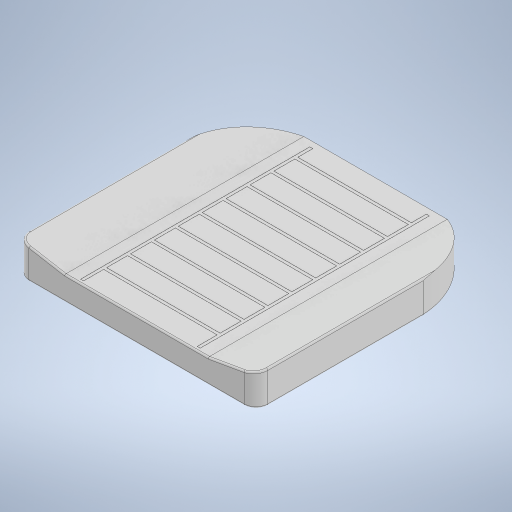
# Autodesk Inventor part: TheSeat(H)
Saved by Autodesk Inventor 2023 (Build 270158030, 158C)
## iProperties
Created: 2023-03-04
Part Number: TheSeat(H)
Material: Generic
Document SubType Name: Modeling
Designer: mpino
Density: 1 g/cm^3
Appearance: Default
Author: mpino
Autodesk Inventor part; units mm, degrees
ref_plane "YZ Plane" through (0, 0, 0) normal (1, 0, 0) x (0, 1, 0)
ref_plane "XZ Plane" through (0, 0, 0) normal (0, 1, 0) x (-1, 0, 0)
ref_plane "XY Plane" through (0, 0, 0) normal (0, 0, 1) x (1, 0, 0)
sketch "Sketch1" plane through (0, 0, 0) normal (0, 1, 0) x (-1, 0, 0)
  line L0 (0, 0) -> (508, 0)
  line L1 (508, 0) -> (508, -508)
  line L2 (508, -508) -> (0, -508)
  line L3 (0, -508) -> (0, 0)
  dimension "d0" = 508
  dimension "d1" = 508
  constraints: 8 end point, 2 parallel, 1 horizontal, 1 perpendicular
  measures "d0" distance of L1.end L2.end
  measures "d1" distance of L0.end L1.end
extrude "Extrusion1" add sketch "Sketch1" along normal blind 50.8
sketch "Sketch2" plane through (0, 50.8, 0) normal (0, 1, 0) x (1, 0, 0)
  line L0 (-508, 0) -> (0, 0) projected
  line L1 (0, 0) -> (0, 25.4)
  line L2 (0, 0) -> (-25.4, 0)
  arc A0 (-25.4, 0) -> (0, 25.4) centre (-25.4, 25.4) ccw
  line L3 (-508, 0) -> (-482.6, 0)
  line L4 (-482.6, 0) -> (-508, 0)
  line L5 (-508, 0) -> (-508, 25.4)
  arc A1 (-508, 25.4) -> (-482.6, 0) centre (-482.6, 25.4) ccw
  line L6 (0, 508) -> (0, 355.6)
  line L7 (0, 508) -> (-101.6, 508)
  arc A2 (0, 355.6) -> (-101.6, 508) centre (-177.6045, 347.2637) ccw
  line L8 (-508, 508) -> (-406.4, 508)
  line L9 (-508, 508) -> (-508, 355.6)
  arc A3 (-406.4, 508) -> (-508, 355.6) centre (-330.3955, 347.2637) ccw
  line L10 (0, 508) -> (-508, 508) projected
  point P0 (-7.4395, 7.4395)
  dimension "d11" = 25.4
  dimension "d12" = 25.4
  dimension "d13" = 25.4
  dimension "d14" = 25.4
  dimension "d81" = 152.4
  dimension "d83" = 177.8
  dimension "d85" = 152.4
  dimension "d86" = 177.8
  dimension "d88" = 7.4395
  dimension "d91" = 101.6
  dimension "d92" = 101.6
  constraints: 18 end point, 9 point on circle, 4 centre point, 4 point on line, 3 tangent, 2 vertical, 1 collinear
  measures "d11" distance of L0.end L1.end
  measures "d12" distance of L0.end L2.end
  measures "d13" distance of L0.start L3.end
  measures "d14" distance of L0.start L5.end
  measures "d81" distance of L6.start L6.end
  measures "d83" radius of A2
  measures "d85" distance of L8.start L9.end
  measures "d86" radius of A3
  measures "d88" distance from line of L1 point (-7.439, 7.439)
  measures "d91" distance of L6.start L7.end
  measures "d92" distance of L8.start L8.end
extrude "Extrusion2" cut sketch "Sketch2" against normal blind 50.8
sketch "Sketch3" plane through (0, 50.8, 0) normal (0, 1, 0) x (1, 0, 0)
  line L0 (0, 0) -> (-254, 0)
  line L1 (-127, 0) -> (-127, 495.3)
  line L2 (-127, 495.3) -> (-133.35, 495.3)
  line L3 (-133.35, 495.3) -> (-133.35, 0)
  line L4 (-381, 0) -> (-381, 495.3)
  line L5 (-381, 495.3) -> (-374.65, 495.3)
  line L6 (-374.65, 495.3) -> (-374.65, 0)
  line L7 (-127, 8.255) -> (-133.35, 8.255)
  line L8 (-374.65, 8.255) -> (-381, 8.255)
  line L9 (-101.6, 508) -> (-406.4, 508) projected
  point P0 (-130.175, 495.3)
  point P1 (-377.825, 495.3)
  dimension "d18" = 254
  dimension "d19" = 127
  dimension "d20" = 6.35
  dimension "d21" = 127
  dimension "d22" = 6.35
  dimension "d34" = 90
  dimension "d35" = 90
  dimension "d36" = 247.65
  dimension "d37" = 8.255
  dimension "d39" = 127
  dimension "d41" = 8.255
  dimension "d42" = 0
  dimension "d43" = 0
  dimension "d89" = 12.7
  dimension "d90" = 12.7
  constraints: 18 end point, 5 parallel, 4 point on line, 2 midpoint, 1 perpendicular, 1 vertical
  measures "d18" distance of L0.start L0.end
  measures "d19" distance of L0.end L1.start
  measures "d20" distance of L1.end L2.end
  measures "d21" distance of L0.end L4.start
  measures "d22" distance of L4.end L5.end
  measures "d34" angle of L5 L1
  measures "d35" angle of L1 L8
  measures "d36" distance between parallel lines of L1 L6
  measures "d37" distance between parallel lines of L7 L0
  measures "d39" distance from line of L0.start L1
  measures "d41" distance from line of L0.start L8
  measures "d42" distance from line of L3.end L0
  measures "d43" distance from line of L6.end L0
  measures "d89" distance from line of L9 point (-130.175, 495.3)
  measures "d90" distance from line of L9 point (-377.825, 495.3)
extrude "Extrusion3" cut sketch "Sketch3" against normal blind 0.254 contours L7 L3 L2 L1 | L4 L5 L6 L8
sketch "Sketch4" plane through (0, 50.8, 0) normal (0, 1, 0) x (1, 0, 0)
  line L0 (-374.65, 495.3) -> (-374.65, 8.255) projected
  line L1 (-374.65, 50.8) -> (-133.35, 50.8)
  line L2 (-133.35, 8.255) -> (-133.35, 495.3) projected
  line L3 (-374.65, 57.15) -> (-133.35, 57.15)
  line L4 (-127, 8.255) -> (-133.35, 8.255) projected
  point P0 (0, 0)
  point P1 (-130.175, 8.255)
  dimension "d44" = 42.545
  dimension "d45" = 6.35
  dimension "d46" = 241.3
  dimension "d47" = 48.895
  dimension "d48" = 241.3
  constraints: 4 end point, 3 point on line, 1 horizontal, 1 midpoint, 1 parallel
  measures "d44" distance from line of L1 point (-130.175, 8.255)
  measures "d45" distance between parallel lines of L1 L3
  measures "d46" distance from line of L3.start L2
  measures "d47" distance from line of point (-374.65, 57.15) L4
  measures "d48" distance from line of point (-374.65, 57.15) L2
extrude "Extrusion4" cut sketch "Sketch4" against normal blind 0.254
sketch "Sketch5" plane through (0, 50.8, 0) normal (0, 1, 0) x (1, 0, 0)
  arc A0 (-25.4, 0) -> (0, 25.4) centre (-25.4, 25.4) ccw projected
  arc A1 (-25.4, 0) -> (0, 25.4) centre (-25.4, 25.4) ccw
  arc A2 (-508, 25.4) -> (-482.6, 0) centre (-482.6, 25.4) ccw
  arc A3 (-406.4, 508) -> (-508, 355.6) centre (-330.3955, 347.2637) ccw projected
  line L0 (-101.6, 508) -> (-406.4, 508) projected
  line L1 (-482.6, 0) -> (-25.4, 0) projected
  line L2 (186.8885, 0) -> (-25.4, 0)
  line L3 (0, 25.4) -> (0, 355.6)
  line L4 (-508, 355.6) -> (-508, 25.4) projected
  line L5 (-508, 25.4) -> (-508, 355.6)
  arc A4 (-406.4, 508) -> (-508, 355.6) centre (-330.3955, 347.2637) ccw
  arc A5 (0, 355.6) -> (-101.6, 508) centre (-177.6045, 347.2637) ccw
  arc A6 (0, 355.6) -> (-101.6, 508) centre (-177.6045, 347.2637) ccw projected
  line L6 (-482.6, 0) -> (-406.4, 0)
  line L7 (-406.4, 508) -> (-406.4, 0)
  line L8 (-101.6, 508) -> (-101.6, 0)
  line L9 (-25.4, 0) -> (-101.6, 0)
  dimension "d96" = 25.4
  constraints: 14 end point, 9 point on circle, 4 centre point, 4 tangent, 3 concentric, 2 collinear, 2 perpendicular, 2 point on line, 1 vertical
  measures "d96" radius of A2
extrude "Extrusion5" add sketch "Sketch5" along normal blind 17.78 contours L1 L8 A5 L3 A0 | L1 A2 L4 A3 L7
sketch "Sketch6" plane through (-482.6, 0, 0) normal (0, 0, 1) x (1, 0, 0)
  line L0 (76.2, 0) -> (76.2, 50.8) projected
  line L1 (-25.4, 68.58) -> (-25.4, 0) projected
  line L2 (76.2, 50.8) -> (-25.4, 68.58)
  line L3 (-25.4, 68.58) -> (76.2, 68.58)
  line L4 (76.2, 68.58) -> (76.2, 50.8)
  line L5 (482.6, 0) -> (482.6, 68.58) projected
  line L6 (381, 50.8) -> (482.6, 68.58)
  line L7 (482.6, 68.58) -> (381, 68.58)
  line L8 (381, 68.58) -> (381, 50.8)
  constraints: 12 end point, 4 perpendicular
extrude "Extrusion6" cut sketch "Sketch6" against normal blind 508
pattern_linear "Rectangular Pattern2" count 11 spacing 50.8 along (0, 0, -1) of "Extrusion4"
sketch "Sketch7" plane through (0, 0, 0) normal (0, -1, 0) x (1, 0, 0)
  line L0 (-171.45, -254) -> (-336.55, -254)
  line L1 (-336.55, -254) -> (-336.55, -76.2)
  line L2 (-336.55, -76.2) -> (-171.45, -76.2)
  line L3 (-171.45, -76.2) -> (-171.45, -254)
  line L4 (-171.45, -254) -> (-336.55, -76.2) construction
  line L5 (-336.55, -254) -> (-171.45, -76.2) construction
  line L6 (-171.45, -76.2) -> (-171.45, -88.9)
  line L7 (-336.55, -76.2) -> (-336.55, -88.9)
  line L8 (-171.45, -254) -> (-184.15, -254)
  line L9 (-184.15, -254) -> (-184.15, -241.3)
  line L10 (-336.55, -254) -> (-323.85, -254)
  line L11 (-323.85, -254) -> (-323.85, -241.3)
  line L12 (-336.55, -88.9) -> (-323.85, -88.9)
  line L13 (-171.45, -88.9) -> (-184.15, -88.9)
  line L14 (-508, -355.6) -> (-508, -25.4) projected
  line L15 (-482.6, 0) -> (-25.4, 0) projected
  line L16 (-336.55, -76.2) -> (-336.55, -50.8)
  line L17 (-171.45, -76.2) -> (-171.45, -50.8)
  line L18 (-171.45, -50.8) -> (-171.45, -25.4)
  line L19 (-171.45, -25.4) -> (-184.15, -25.4)
  line L20 (-171.45, -50.8) -> (-184.15, -50.8)
  line L21 (-133.35, -50.8) -> (-374.65, -50.8) projected
  line L22 (-336.55, -76.2) -> (-336.55, -25.4)
  line L23 (-336.55, -25.4) -> (-323.85, -25.4)
  line L24 (-336.55, -50.8) -> (-323.85, -50.8)
  point P0 (-254, -165.1)
  point P1 (-254, 0)
  point P2 (-330.2, -25.4)
  dimension "d58" = 165.1
  dimension "d59" = 177.8
  dimension "d60" = 12.7
  dimension "d63" = 12.7
  dimension "d65" = 12.7
  dimension "d66" = 12.7
  dimension "d67" = 12.7
  dimension "d69" = 12.7
  dimension "d78" = 12.7
  dimension "d79" = 12.7
  dimension "d98" = 254
  dimension "d99" = 165.1
  dimension "d100" = 25.4
  dimension "d101" = 25.4
  dimension "d102" = 25.4
  dimension "d103" = 12.7
  dimension "d104" = 12.7
  dimension "d105" = 12.7
  dimension "d106" = 12.7
  dimension "d107" = 25.4
  constraints: 44 end point, 7 point on line, 5 perpendicular, 4 midpoint, 3 horizontal, 3 vertical, 2 parallel
  measures "d58" distance of L1.end L2.end
  measures "d59" distance of L0.end L1.end
  measures "d60" distance of L2.end L6.end
  measures "d63" distance of L1.end L7.end
  measures "d65" distance of L0.start L8.end
  measures "d66" distance of L8.end L9.end
  measures "d67" distance of L0.end L10.end
  measures "d69" distance of L10.end L11.end
  measures "d78" distance of L7.end L12.end
  measures "d79" distance of L6.end L13.end
  measures "d98" distance from line of L14 point (-254, -165.1)
  measures "d99" distance of point (-254, 0) point (-254, -165.1)
  measures "d100" distance of L1.end L16.end
  measures "d101" distance of L2.end L17.end
  measures "d102" distance of L17.end L18.end
  measures "d103" distance of L18.end L19.end
  measures "d104" distance of L17.end L20.end
  measures "d105" distance of L22.end L23.end
  measures "d106" distance of L16.end L24.end
  measures "d107" distance from line of L15 point (-330.2, -25.4)
hole "Hole1" at (-184.15, 0, -241.3) at (-323.85, 0, -241.3) at (-323.85, 0, -88.9) at (-184.15, 0, -88.9) at (-184.15, 0, -50.8) at (-184.15, 0, -25.4) at (-323.85, 0, -25.4) at (-323.85, 0, -50.8) direction (0, 1, 0) diameter 4.9784 depth 19.05 tip angle 118 thread size "1/4-20 UNC" class "2B" standard "ANSI Unified Screw Threads"
fillet "Fillet3" radius 3.175 11 edges at (-29.6659, 0, -445.8894) (-254, 0, -508) (-478.3341, 0, -445.8894) (-500.5605, 0, -7.4395) (-254, 0, 0) (-7.4395, 0, -7.4395) (0, 0, -190.5) (-508, 0, -190.5) (0, 68.58, -190.5) (-254, 50.8, 0) (-508, 68.58, -190.5)
body "Solid1"
